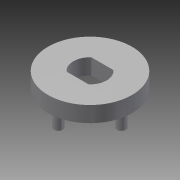
# Autodesk Inventor part: P60 Carrier Plate (output)
Saved by Autodesk Inventor 2014 SP1 (Build 180222100, 222)
## iProperties
Created: 2013-05-05
Part Number: P60 Carrier Plate (output)
Material: Steel
Document SubType Name: Modeling
Designer: Moses
Density: 7.85 g/cm^3
Mass: 14.6073 g
Surface Area: 14.0901 cm^2
Volume: 1.86081 cm^3
Appearance: Steel
Author: Moses
Autodesk Inventor part; units mm, degrees
ref_plane "YZ Plane" through (0, 0, 0) normal (1, 0, 0) x (0, 1, 0)
ref_plane "XZ Plane" through (0, 0, 0) normal (0, 1, 0) x (-1, 0, 0)
ref_plane "XY Plane" through (0, 0, 0) normal (0, 0, 1) x (1, 0, 0)
sketch "Sketch1" plane through (0, 0, 0) normal (0, 1, 0) x (-1, 0, 0)
  circle A0 centre (0, 0) radius 12
  arc A1 (-0.484, 4.4186) -> (-1.3551, 4.2334) centre (0, 0) ccw construction
  arc A2 (-2.3154, 4.5441) -> (-2.0424, 3.145) centre (1.9294, 4.6461) ccw construction
  arc A3 (-2.0424, 3.145) -> (-2.36, 2.9143) centre (0, 0) ccw construction
  arc A4 (-2.36, 2.9143) -> (-3.6062, 3.6062) centre (-5.0149, -0.3993) ccw construction
  arc A5 (-3.6062, 3.6062) -> (-3.9634, 3.2095) centre (0, 0) ccw construction
  arc A6 (-3.9634, 3.2095) -> (-3.145, 2.0424) centre (-0.1271, 5.0291) ccw construction
  arc A7 (-3.145, 2.0424) -> (-3.3413, 1.7025) centre (0, 0) ccw construction
  arc A8 (-3.3413, 1.7025) -> (-4.7613, 1.8277) centre (-4.4189, -2.4045) ccw construction
  arc A9 (-4.7613, 1.8277) -> (-4.9262, 1.32) centre (0, 0) ccw construction
  arc A10 (-4.9262, 1.32) -> (-3.7038, 0.5866) centre (-2.1617, 4.5426) ccw construction
  arc A11 (-3.7038, 0.5866) -> (-3.7449, 0.1963) centre (0, 0) ccw construction
  arc A12 (-3.7449, 0.1963) -> (-5.093, -0.2669) centre (-3.0589, -3.9939) ccw construction
  arc A13 (-5.093, -0.2669) -> (-5.0372, -0.7978) centre (0, 0) ccw construction
  arc A14 (-5.0372, -0.7978) -> (-3.6222, -0.9706) centre (-3.8224, 3.2707) ccw construction
  arc A15 (-3.6222, -0.9706) -> (-3.5009, -1.3439) centre (0, 0) ccw construction
  arc A16 (-3.5009, -1.3439) -> (-4.5441, -2.3154) centre (-1.17, -4.8928) ccw construction
  arc A17 (-4.5441, -2.3154) -> (-4.2772, -2.7777) centre (0, 0) ccw construction
  arc A18 (-4.2772, -2.7777) -> (-2.9143, -2.36) centre (-4.8223, 1.4332) ccw construction
  arc A19 (-2.9143, -2.36) -> (-2.6517, -2.6517) centre (0, 0) ccw construction
  arc A20 (-2.6517, -2.6517) -> (-3.2095, -3.9634) centre (0.9213, -4.9457) ccw construction
  arc A21 (-3.2095, -3.9634) -> (-2.7777, -4.2772) centre (0, 0) ccw construction
  arc A22 (-2.7777, -4.2772) -> (-1.7025, -3.3413) centre (-4.9883, -0.6521) ccw construction
  arc A23 (-1.7025, -3.3413) -> (-1.3439, -3.5009) centre (0, 0) ccw construction
  arc A24 (-1.3439, -3.5009) -> (-1.32, -4.9262) centre (2.8532, -4.1434) ccw construction
  arc A25 (-1.32, -4.9262) -> (-0.7978, -5.0372) centre (0, 0) ccw construction
  arc A26 (-0.7978, -5.0372) -> (-0.1963, -3.7449) centre (-4.2918, -2.6247) ccw construction
  arc A27 (-0.1963, -3.7449) -> (0.1963, -3.7449) centre (0, 0) ccw construction
  arc A28 (0.1963, -3.7449) -> (0.7978, -5.0372) centre (4.2918, -2.6247) ccw construction
  arc A29 (0.7978, -5.0372) -> (1.32, -4.9262) centre (0, 0) ccw construction
  arc A30 (1.32, -4.9262) -> (1.3439, -3.5009) centre (-2.8532, -4.1434) ccw construction
  arc A31 (1.3439, -3.5009) -> (1.7025, -3.3413) centre (0, 0) ccw construction
  arc A32 (1.7025, -3.3413) -> (2.7777, -4.2772) centre (4.9883, -0.6521) ccw construction
  arc A33 (2.7777, -4.2772) -> (3.2095, -3.9634) centre (0, 0) ccw construction
  arc A34 (3.2095, -3.9634) -> (2.6517, -2.6517) centre (-0.9213, -4.9457) ccw construction
  arc A35 (2.6517, -2.6517) -> (2.9143, -2.36) centre (0, 0) ccw construction
  arc A36 (2.9143, -2.36) -> (4.2772, -2.7777) centre (4.8223, 1.4332) ccw construction
  arc A37 (4.2772, -2.7777) -> (4.5441, -2.3154) centre (0, 0) ccw construction
  arc A38 (4.5441, -2.3154) -> (3.5009, -1.3439) centre (1.17, -4.8928) ccw construction
  arc A39 (3.5009, -1.3439) -> (3.6222, -0.9706) centre (0, 0) ccw construction
  arc A40 (3.6222, -0.9706) -> (5.0372, -0.7978) centre (3.8224, 3.2707) ccw construction
  arc A41 (5.0372, -0.7978) -> (5.093, -0.2669) centre (0, 0) ccw construction
  arc A42 (5.093, -0.2669) -> (3.7449, 0.1963) centre (3.0589, -3.9939) ccw construction
  arc A43 (3.7449, 0.1963) -> (3.7038, 0.5866) centre (0, 0) ccw construction
  arc A44 (3.7038, 0.5866) -> (4.9262, 1.32) centre (2.1617, 4.5426) ccw construction
  arc A45 (4.9262, 1.32) -> (4.7613, 1.8277) centre (0, 0) ccw construction
  arc A46 (4.7613, 1.8277) -> (3.3413, 1.7025) centre (4.4189, -2.4045) ccw construction
  arc A47 (3.3413, 1.7025) -> (3.145, 2.0424) centre (0, 0) ccw construction
  arc A48 (3.145, 2.0424) -> (3.9634, 3.2095) centre (0.1271, 5.0291) ccw construction
  arc A49 (3.9634, 3.2095) -> (3.6062, 3.6062) centre (0, 0) ccw construction
  arc A50 (3.6062, 3.6062) -> (2.36, 2.9143) centre (5.0149, -0.3993) ccw construction
  arc A51 (2.36, 2.9143) -> (2.0424, 3.145) centre (0, 0) ccw construction
  arc A52 (2.0424, 3.145) -> (2.3154, 4.5441) centre (-1.9294, 4.6461) ccw construction
  arc A53 (2.3154, 4.5441) -> (1.8277, 4.7613) centre (0, 0) ccw construction
  arc A54 (1.8277, 4.7613) -> (0.9706, 3.6222) centre (4.7437, 1.675) ccw construction
  arc A55 (0.9706, 3.6222) -> (0.5866, 3.7038) centre (0, 0) ccw construction
  arc A56 (0.5866, 3.7038) -> (0.2669, 5.093) centre (-3.6523, 3.4596) ccw construction
  arc A57 (0.2669, 5.093) -> (-0.2669, 5.093) centre (0, 0) ccw construction
  arc A58 (-0.2669, 5.093) -> (-0.5866, 3.7038) centre (3.6523, 3.4596) ccw construction
  arc A59 (-0.5866, 3.7038) -> (-0.9706, 3.6222) centre (0, 0) ccw construction
  arc A60 (-0.9706, 3.6222) -> (-1.8277, 4.7613) centre (-4.7437, 1.675) ccw construction
  arc A61 (-1.8277, 4.7613) -> (-2.3154, 4.5441) centre (0, 0) ccw construction
  circle A62 centre (0, 0) radius 1.25 construction
  arc A63 (0.484, 4.4186) -> (-0.484, 4.4186) centre (0, 0) ccw construction
  arc A64 (1.3551, 4.2334) -> (0.484, 4.4186) centre (0, 0) ccw construction
  arc A65 (2.2393, 3.8397) -> (1.3551, 4.2334) centre (0, 0) ccw construction
  arc A66 (2.9598, 3.3163) -> (2.2393, 3.8397) centre (0, 0) ccw construction
  arc A67 (3.6075, 2.597) -> (2.9598, 3.3163) centre (0, 0) ccw construction
  arc A68 (4.0528, 1.8257) -> (3.6075, 2.597) centre (0, 0) ccw construction
  arc A69 (4.3519, 0.9051) -> (4.0528, 1.8257) centre (0, 0) ccw construction
  arc A70 (4.445, 0.0194) -> (4.3519, 0.9051) centre (0, 0) ccw construction
  arc A71 (4.3438, -0.9432) -> (4.445, 0.0194) centre (0, 0) ccw construction
  arc A72 (4.0686, -1.7902) -> (4.3438, -0.9432) centre (0, 0) ccw construction
  arc A73 (3.5846, -2.6284) -> (4.0686, -1.7902) centre (0, 0) ccw construction
  arc A74 (2.9887, -3.2902) -> (3.5846, -2.6284) centre (0, 0) ccw construction
  arc A75 (2.2056, -3.8592) -> (2.9887, -3.2902) centre (0, 0) ccw construction
  arc A76 (1.3921, -4.2214) -> (2.2056, -3.8592) centre (0, 0) ccw construction
  arc A77 (0.4453, -4.4226) -> (1.3921, -4.2214) centre (0, 0) ccw construction
  arc A78 (-0.4453, -4.4226) -> (0.4453, -4.4226) centre (0, 0) ccw construction
  arc A79 (-1.3921, -4.2214) -> (-0.4453, -4.4226) centre (0, 0) ccw construction
  arc A80 (-2.2056, -3.8592) -> (-1.3921, -4.2214) centre (0, 0) ccw construction
  arc A81 (-2.9887, -3.2902) -> (-2.2056, -3.8592) centre (0, 0) ccw construction
  arc A82 (-3.5846, -2.6284) -> (-2.9887, -3.2902) centre (0, 0) ccw construction
  arc A83 (-4.0686, -1.7902) -> (-3.5846, -2.6284) centre (0, 0) ccw construction
  arc A84 (-4.3438, -0.9432) -> (-4.0686, -1.7902) centre (0, 0) ccw construction
  arc A85 (-4.445, 0.0194) -> (-4.3438, -0.9432) centre (0, 0) ccw construction
  arc A86 (-4.3519, 0.9051) -> (-4.445, 0.0194) centre (0, 0) ccw construction
  arc A87 (-4.0528, 1.8257) -> (-4.3519, 0.9051) centre (0, 0) ccw construction
  arc A88 (-3.6075, 2.597) -> (-4.0528, 1.8257) centre (0, 0) ccw construction
  arc A89 (-2.9598, 3.3163) -> (-3.6075, 2.597) centre (0, 0) ccw construction
  arc A90 (-2.2393, 3.8397) -> (-2.9598, 3.3163) centre (0, 0) ccw construction
  arc A91 (-1.3551, 4.2334) -> (-2.2393, 3.8397) centre (0, 0) ccw construction
  circle A92 centre (0, 0) radius 9 construction
  circle A93 centre (0, 9) radius 1.25
  line L0 (0, 9) -> (0, 0) construction
  circle A94 centre (-9, 0) radius 1.25
  circle A95 centre (0, -9) radius 1.25
  circle A96 centre (9, 0) radius 1.25
  circle A97 centre (0, 0) radius 4.7625
  line L1 (-3.175, 3.5498) -> (3.175, 3.5498)
  line L2 (-3.175, -3.5498) -> (3.175, -3.5498)
  dimension "d1" = 8.89
  dimension "d2" = 18
  dimension "d3" = 24
  dimension "d4" = 2.5
  dimension "d7" = 360
  dimension "d13" = 9.525
  dimension "d14" = 6.35
  constraints: 154 point on circle, 67 centre point, 6 end point, 2 coincident, 2 horizontal alignment, 2 parallel, 1 perpendicular, 1 vertical, 1 vertical alignment, 283 other
  measures "d3" diameter of A0
  measures "d4" diameter of A93
  measures "d13" diameter of A97
  measures "d14" distance of L1.start L1.end
extrude "Extrusion1" add sketch "Sketch1" along normal blind 4.5 contours A0 | A93 | A94 | A95 | A96 | L1 A97 | A97 L2
extrude "Extrusion2" add sketch "Sketch1" against normal blind 5 contours A93 | A94 | A95 | A96
body "Solid1"
